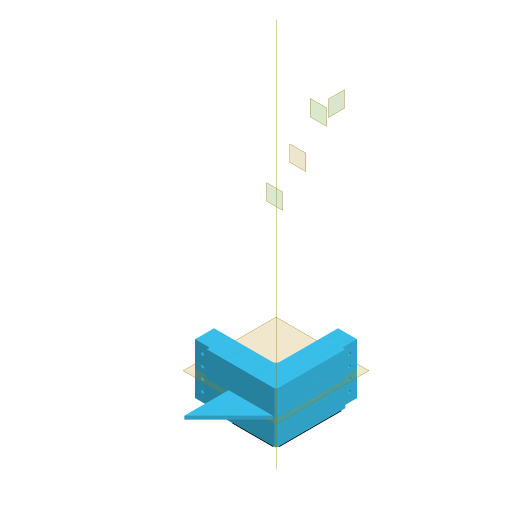
# Autodesk Inventor part: Столбик
Saved by Autodesk Inventor 2023.2 (Build 272271030, 271C)
## iProperties
Created: 2025-04-23
Part Number: Столбик
Material: Типовые
Document SubType Name: Modeling
Designer: Коноваленко
Density: 1 g/cm^3
Appearance: Бирюзовый
Author: Коноваленко
Autodesk Inventor part; units mm, degrees
ref_plane "YZ Plane" through (0, 0, 0) normal (1, 0, 0) x (0, 1, 0)
ref_plane "XY Plane" through (0, 0, 0) normal (0, 0, 1) x (1, 0, 0)
sketch "Эскиз1" plane through (0, 0, 0) normal (0, 1, 0) x (-1, 0, 0)
  line L0 (-30, -85) -> (-30, 30)
  line L1 (-30, 30) -> (85, 30)
  line L2 (85, 30) -> (85, 0)
  line L3 (85, 0) -> (0, 0)
  line L4 (0, 0) -> (0, -85)
  line L5 (0, -85) -> (-30, -85)
  circle A0 centre (-26, 26) radius 4
  line L6 (85, 26) -> (65, 26)
  line L7 (65, 26) -> (65, 30)
  circle A1 centre (5, -5) radius 5
  line L8 (-30, -85) -> (-26, -85)
  line L9 (-26, -85) -> (-26, -65)
  line L10 (-26, -65) -> (-30, -65)
  line L11 (-30, -65) -> (-30, -85)
  line L12 (0, -85) -> (-4, -85)
  line L13 (0, -65) -> (0, -85)
  line L14 (85, 0) -> (65, 0)
  line L15 (85, 4) -> (85, 0)
  point P0 (-26, 30)
  point P1 (-30, 26)
  point P2 (0, -5)
  point P3 (5, 0)
  dimension "d0" = 115
  dimension "d1" = 115
  dimension "d2" = 30
  dimension "d3" = 30
  dimension "d6" = 4
  dimension "d7" = 20
  dimension "d8" = 10
  dimension "d9" = 4
  dimension "d10" = 20
  dimension "d26" = 8
  constraints: 32 end point, 7 perpendicular, 4 horizontal, 4 point on line, 4 tangent, 2 centre point, 2 parallel, 1 vertical
  measures "d0" distance of L0.end L1.end
  measures "d1" distance of L0.start L0.end
  measures "d2" distance between parallel lines of L1 L3
  measures "d3" distance between parallel lines of L0 L4
  measures "d6" distance between parallel lines of L6 L1
  measures "d7" distance between parallel lines of L2 L7
  measures "d8" diameter of A1
  measures "d9" distance between parallel lines of L0 L9
  measures "d10" distance of L8.end L9.end
  measures "d26" diameter of A0
extrude "Выдавливание1" add sketch "Эскиз1" along normal blind 70 contours L0 A0 L1 L7 L6 L2 L3 L4 L5 L9 L10 | A0 | L4 L3 A1
sketch "Эскиз2" plane through (0, 0, 0) normal (0, -1, 0) x (1, 0, 0)
  line L0 (-5, 0) -> (-85, 0) projected
  line L1 (-30, 0) -> (-30, 30)
  line L2 (-30, 30) -> (26, 30)
  line L3 (30, 26) -> (30, -59)
  line L4 (0, -85) -> (0, -5) projected
  arc A0 (0, -5) -> (-5, 0) centre (-5, -5) ccw projected
  line L5 (0, -85) -> (0, -5) projected
  arc A1 (30, 26) -> (26, 30) centre (26, 26) ccw projected
  line L6 (30, -59) -> (0, -59)
  point P0 (0, 0)
  point P1 (-30, 15)
  point P2 (-65, 0)
  point P3 (0, -65)
  point P4 (0, -59)
  dimension "d134" = 60
  dimension "d135" = 30
  dimension "d136" = 30
  dimension "d137" = 85
  constraints: 8 end point, 4 perpendicular, 2 point on circle, 2 point on line, 1 midpoint
  measures "d134" distance between parallel lines of L3 L1
  measures "d135" distance between parallel lines of L0 L2
  measures "d136" distance between parallel lines of L4 L3
  measures "d137" distance of L3.start L3.end
sketch "Эскиз13" plane through (0, 70, 0) normal (0, 1, 0) x (1, 0, 0)
  line L0 (26, 65) -> (26, 85) projected
  line L1 (26, 85) -> (0, 85) projected
  line L2 (30, 65) -> (26, 65) projected
  line L3 (0, 30) -> (30, 30)
  line L4 (30, -26) -> (30, 65) projected
  line L5 (0, 85) -> (0, 5) projected
  point P0 (0, 0)
  point P1 (30, -30)
  dimension "d226" = 55
  constraints: 2 end point, 1 horizontal, 1 point on line
  measures "d226" distance between parallel lines of L1 L3
extrude "Выдавливание11" [suppressed]
ref_plane "РабПлоскость2" through (0, 300, -30) normal (0, 0, 1) x (1, 0, 0)
sketch "Эскиз16" plane through (0, 300, -30) normal (0, 0, 1) x (1, 0, 0)
  line L0 (7.5, 7) -> (22.5, 7)
  line L1 (22.5, 7) -> (20, 0)
  line L2 (7.5, 7) -> (10, 0)
  line L3 (30, -230) -> (30, 70) projected
  line L4 (10, 0) -> (20, 0)
  line L5 (30, -230) -> (30, 70) projected
  line L6 (0, 144) -> (0, -374) projected
  line L7 (30, -300) -> (30, -230) projected
  point P0 (96.6667, 0)
  dimension "d143" = 15
  dimension "d207" = 7
  dimension "d222" = 10
  dimension "d223" = 7.5
  dimension "d224" = 10
  constraints: 8 end point, 2 horizontal, 1 point on line
  measures "d143" distance of L0.start L0.end
  measures "d207" distance between parallel lines of L0 L4
  measures "d222" distance from line of L6 L2.end
  measures "d223" distance from line of L7 L0.end
  measures "d224" distance from line of L7 L1.end
extrude "Выдавливание13" [suppressed]
feature "Оболочка1" [suppressed]
fillet "Сопряжение6" [suppressed]
fillet "Сопряжение8" [suppressed]
sketch "Эскиз28" plane through (-80, 5, 0) normal (0, 1, 0) x (1, 0, 0)
  arc A0 (103, -25) -> (105, -23) centre (103, -23) ccw projected
  line L0 (105, -23) -> (105, 58) projected
  arc A1 (105, 58) -> (103, 60) centre (103, 58) ccw projected
  arc A2 (101, 62) -> (103, 60) centre (103, 62) ccw projected
  line L1 (101, 62) -> (101, 78) projected
  arc A3 (101, 78) -> (99, 80) centre (99, 78) ccw projected
  line L2 (99, 80) -> (80, 80) projected
  line L3 (80, 5) -> (80, 80) projected
  arc A4 (75, 0) -> (80, 5) centre (75, 5) ccw projected
  line L4 (0, 0) -> (75, 0) projected
  line L5 (0, 0) -> (0, -19) projected
  arc A5 (0, -19) -> (2, -21) centre (2, -19) ccw projected
  line L6 (2, -21) -> (18, -21) projected
  arc A6 (20, -23) -> (18, -21) centre (18, -23) ccw projected
  arc A7 (20, -23) -> (22, -25) centre (22, -23) ccw projected
  line L7 (22, -25) -> (103, -25) projected
  point P0 (80, 0)
extrude "Выдавливание19" [suppressed]
sketch "Эскиз27" plane through (-60, 10, 25) normal (0, 1, 0) x (1, 0, 0)
  circle A0 centre (75, 70) radius 3.1
  circle A1 centre (75, 40) radius 3.1
  circle A2 centre (75, 10) radius 3.1
  circle A3 centre (45, 10) radius 3.1
  circle A4 centre (15, 10) radius 3.1
  line L0 (83, 0) -> (2, 0) projected
  dimension "d231" = 17.945
  dimension "d234" = 10
  constraints: 5 centre point, 1 equal radius, 8 other
  measures "d234" distance from line of L0 A4.centre
ref_plane "РабПлоскость3" through (-80, 140, 0) normal (0, 1, 0) x (1, 0, 0)
sketch "Эскиз30" plane through (-80, 140, 0) normal (0, 1, 0) x (1, 0, 0)
  line L0 (103, -25) -> (22, -25) projected
  arc A0 (103, -25) -> (105, -23) centre (103, -23) ccw projected
  line L1 (105, 58) -> (105, -23) projected
  arc A1 (105, 58) -> (103, 60) centre (103, 58) ccw projected
  arc A2 (101, 62) -> (103, 60) centre (103, 62) ccw projected
  line L2 (101, 78) -> (101, 62) projected
  arc A3 (101, 78) -> (99, 80) centre (99, 78) ccw projected
  line L3 (80, 80) -> (99, 80) projected
  line L4 (80, 80) -> (80, 5) projected
  arc A4 (75, 0) -> (80, 5) centre (75, 5) ccw projected
  line L5 (75, 0) -> (0, 0) projected
  line L6 (0, -19) -> (0, 0) projected
  arc A5 (0, -19) -> (2, -21) centre (2, -19) ccw projected
  line L7 (18, -21) -> (2, -21) projected
  arc A6 (20, -23) -> (18, -21) centre (18, -23) ccw projected
  arc A7 (20, -23) -> (22, -25) centre (22, -23) ccw projected
  circle A8 centre (65, -15) radius 3.1 projected
  circle A9 centre (35, -15) radius 3.1 projected
  circle A10 centre (95, -15) radius 3.1 projected
  circle A11 centre (95, 15) radius 3.1 projected
  circle A12 centre (95, 45) radius 3.1 projected
  point P0 (80, 0)
extrude "Выдавливание20" [suppressed]
ref_plane "РабПлоскость4" through (-80, 150, 0) normal (0, -1, 0) x (1, 0, 0)
ref_plane "РабПлоскость5" through (-80, 100, 0) normal (0, 1, 0) x (1, 0, 0)
sketch "Эскиз31" plane through (-80, 100, 0) normal (0, 1, 0) x (1, 0, 0)
  arc A0 (103, 60) -> (101, 62) centre (103, 62) ccw projected
  arc A1 (105, 58) -> (103, 60) centre (103, 58) ccw projected
  line L0 (105, -23) -> (105, 58) projected
  arc A2 (103, -25) -> (105, -23) centre (103, -23) ccw projected
  line L1 (22, -25) -> (103, -25) projected
  arc A3 (20, -23) -> (22, -25) centre (22, -23) ccw projected
  arc A4 (18, -21) -> (20, -23) centre (18, -23) ccw projected
  line L2 (2, -21) -> (18, -21) projected
  arc A5 (0, -19) -> (2, -21) centre (2, -19) ccw projected
  line L3 (0, 0) -> (0, -19) projected
  line L4 (75, 0) -> (0, 0) projected
  line L5 (80, 80) -> (80, 5) projected
  line L6 (99, 80) -> (80, 80) projected
  arc A6 (101, 78) -> (99, 80) centre (99, 78) ccw projected
  line L7 (101, 62) -> (101, 78) projected
  arc A7 (75, 0) -> (80, 5) centre (75, 5) ccw projected
  point P0 (80, 0)
  constraints: 7 centre point
extrude "Выдавливание21" [suppressed]
pattern_linear "Прямоуг.массив1" [suppressed]
ref_plane "РабПлоскость8" through (-80, 200, 0) normal (0, 1, 0) x (1, 0, 0)
sketch "Эскиз33" plane through (-80, 200, 0) normal (0, 1, 0) x (1, 0, 0)
  arc A0 (101, 62) -> (103, 60) centre (103, 62) ccw projected
  line L0 (101, 78) -> (101, 62) projected
  line L1 (80, 80) -> (99, 80) projected
  line L2 (80, 80) -> (80, 5) projected
  line L3 (75, 0) -> (0, 0) projected
  line L4 (0, -19) -> (0, 0) projected
  line L5 (18, -21) -> (2, -21) projected
  arc A1 (20, -23) -> (18, -21) centre (18, -23) ccw projected
  line L6 (103, -25) -> (22, -25) projected
  line L7 (105, 58) -> (105, -23) projected
  arc A2 (20, -23) -> (22, -25) centre (22, -23) ccw projected
  arc A3 (20, -23) -> (22, -25) centre (22, -23) ccw projected
  arc A4 (0, -19) -> (2, -21) centre (2, -19) ccw projected
  arc A5 (0, -19) -> (2, -21) centre (2, -19) ccw projected
  arc A6 (103, -25) -> (105, -23) centre (103, -23) ccw projected
  arc A7 (103, -25) -> (105, -23) centre (103, -23) ccw projected
  arc A8 (75, 0) -> (80, 5) centre (75, 5) ccw projected
  arc A9 (101, 78) -> (99, 80) centre (99, 78) ccw projected
  arc A10 (105, 58) -> (103, 60) centre (103, 58) ccw projected
  arc A11 (105, 58) -> (103, 60) centre (103, 58) ccw projected
  arc A12 (20, -23) -> (22, -25) centre (22, -23) ccw projected
  arc A13 (20, -23) -> (22, -25) centre (22, -23) ccw projected
  arc A14 (20, -23) -> (22, -25) centre (22, -23) ccw projected
  arc A15 (20, -23) -> (22, -25) centre (22, -23) ccw projected
  arc A16 (20, -23) -> (22, -25) centre (22, -23) ccw projected
  arc A17 (20, -23) -> (22, -25) centre (22, -23) ccw projected
  arc A18 (0, -19) -> (2, -21) centre (2, -19) ccw projected
  arc A19 (0, -19) -> (2, -21) centre (2, -19) ccw projected
  arc A20 (0, -19) -> (2, -21) centre (2, -19) ccw projected
  arc A21 (0, -19) -> (2, -21) centre (2, -19) ccw projected
  arc A22 (0, -19) -> (2, -21) centre (2, -19) ccw projected
  arc A23 (0, -19) -> (2, -21) centre (2, -19) ccw projected
  arc A24 (103, -25) -> (105, -23) centre (103, -23) ccw projected
  arc A25 (103, -25) -> (105, -23) centre (103, -23) ccw projected
  arc A26 (103, -25) -> (105, -23) centre (103, -23) ccw projected
  arc A27 (103, -25) -> (105, -23) centre (103, -23) ccw projected
  arc A28 (103, -25) -> (105, -23) centre (103, -23) ccw projected
  arc A29 (103, -25) -> (105, -23) centre (103, -23) ccw projected
  arc A30 (101, 78) -> (99, 80) centre (99, 78) ccw projected
  arc A31 (101, 78) -> (99, 80) centre (99, 78) ccw projected
  arc A32 (101, 78) -> (99, 80) centre (99, 78) ccw projected
  arc A33 (101, 78) -> (99, 80) centre (99, 78) ccw projected
  arc A34 (101, 78) -> (99, 80) centre (99, 78) ccw projected
  arc A35 (101, 78) -> (99, 80) centre (99, 78) ccw projected
  arc A36 (101, 78) -> (99, 80) centre (99, 78) ccw projected
  arc A37 (105, 58) -> (103, 60) centre (103, 58) ccw projected
  arc A38 (105, 58) -> (103, 60) centre (103, 58) ccw projected
  arc A39 (105, 58) -> (103, 60) centre (103, 58) ccw projected
  arc A40 (105, 58) -> (103, 60) centre (103, 58) ccw projected
  arc A41 (105, 58) -> (103, 60) centre (103, 58) ccw projected
  arc A42 (105, 58) -> (103, 60) centre (103, 58) ccw projected
  point P0 (80, 0)
  point P1 (2, -21)
  point P2 (20, -23)
  point P3 (22, -25)
  constraints: 2 centre point
extrude "Выдавливание24" [suppressed]
pattern_linear "Прямоуг.массив2" [suppressed]
feature "Разделение3" [suppressed]
fillet "Сопряжение9" [suppressed]
fillet "Сопряжение10" [suppressed]
extrude "Выдавливание25" [suppressed]
ref_plane "РабПлоскость13" through (23, 363, -35) normal (0, 0, -1) x (-1, 0, 0)
sketch "Эскиз34" plane through (23, 363, -35) normal (0, 0, -1) x (-1, 0, 0)
  line L0 (7.595, -61) -> (8, -62.1339) projected
  line L1 (7.595, -61) -> (8, -62.1339) projected
  line L2 (8.405, -61) -> (7.595, -61) projected
  line L3 (8, -62.1339) -> (8.405, -61) projected
  point P0 (23, -363)
extrude "Выдавливание26" [suppressed]
sketch "Эскиз36" plane through (25, 57, 23) normal (-1, 0, 0) x (0, 0, 1)
  line L0 (-28, 38) -> (-101, 38) projected
  line L1 (-101, -2) -> (-28, -2) projected
  line L2 (-76, 38) -> (-71, 38)
  line L3 (-71, 38) -> (-71, -2)
  line L4 (-71, -2) -> (-76, -2)
  line L5 (-76, -2) -> (-76, 38)
  line L6 (-81, 0) -> (-81, 36) projected
  point P0 (-23, -57)
  point P1 (-76, -2)
  dimension "d264" = 14.559
  dimension "d270" = 5.467
  constraints: 8 end point, 2 parallel, 2 point on line, 1 horizontal, 1 perpendicular
extrude "Выдавливание27" [suppressed]
pattern_linear "Прямоуг.массив3" [suppressed]
ref_plane "РабПлоскость10" through (-85, 0, -85) normal (0.7071068, 0, -0.7071068) x (0, -1, 0)
mirror "Зеркальное отражение9" [suppressed]
ref_plane "РабПлоскость12" through (23, 293, 25) normal (0, 0, -1) x (-1, 0, 0)
sketch "Эскиз38" plane through (23, 293, 25) normal (0, 0, -1) x (-1, 0, 0)
  line L0 (64.282, 2) -> (76, 2)
  line L1 (76, 2) -> (76, -43)
  line L2 (76, -43) -> (64.282, -43)
  line L3 (64.282, -43) -> (64.282, 2)
  line L4 (83, 2) -> (85, 2) projected
  line L5 (81, 2) -> (81, -41) projected
  line L6 (28, -43) -> (101, -43) projected
  point P0 (23, -293)
  point P1 (84, 2)
  point P2 (70.141, -43)
  dimension "d279" = 11.718
  dimension "d301" = 5
  constraints: 8 end point, 2 midpoint, 2 parallel, 2 point on line, 1 horizontal, 1 perpendicular
  measures "d279" distance between parallel lines of L3 L1
  measures "d301" distance between parallel lines of L5 L1
extrude "Выдавливание29" [suppressed]
ref_plane "РабПлоскость11" through (25, 363, -58) normal (-1, 0, 0) x (0, 0, 1)
sketch "Эскиз40" plane through (25, 295, -35) normal (-1, 0, 0) x (0, 0, 1)
  line L0 (0, 0) -> (30, 0) projected
  line L1 (-23, -45) -> (58, -45) projected
  line L2 (-45, 70) -> (0, 70) projected
  line L3 (-18, 70) -> (-13, 70)
  line L4 (-13, -45) -> (-18, -45)
  line L5 (-45, 70) -> (-45, -43) projected
  line L6 (0, 0) -> (0, 70) projected
  line L7 (0, 40) -> (0, 35)
  line L8 (-45, 35) -> (-45, 40)
  line L9 (-45, 5) -> (-45, 0)
  line L10 (0, 0) -> (0, 5)
  line L11 (12, 0) -> (17, 0)
  line L12 (17, 0) -> (17, -45)
  line L13 (17, -45) -> (12, -45)
  line L14 (12, -45) -> (12, 0)
  line L15 (-43, -45) -> (30, -45) projected
  line L16 (-45, 40) -> (-18, 40)
  line L17 (-13, 40) -> (0, 40)
  line L18 (-18, 40) -> (-18, 70)
  line L19 (0, 35) -> (-13, 35)
  line L20 (-18, 35) -> (-45, 35)
  line L21 (-13, 70) -> (-13, 40)
  line L22 (0, 5) -> (-13, 5)
  line L23 (-18, 5) -> (-45, 5)
  line L24 (-18, -45) -> (-18, 0)
  line L25 (-18, 5) -> (-18, 35)
  line L26 (-45, 0) -> (-18, 0)
  line L27 (-13, 0) -> (0, 0)
  line L28 (-13, 35) -> (-13, 5)
  line L29 (-13, 0) -> (-13, -45)
  point P0 (35, -295)
  point P1 (15, 0)
  point P2 (14.5, -45)
  point P3 (12, 0)
  point P4 (17, 0)
  point P5 (-45, 5)
  point P6 (-45, 0)
  point P7 (-18, -45)
  point P8 (-13, -45)
  point P9 (0, 40)
  point P10 (-13, 70)
  point P11 (-45, 35)
  dimension "d312" = 7.296
  dimension "d313" = 53.553
  dimension "d314" = 30
  dimension "d315" = 13
  dimension "d316" = 5
  dimension "d317" = 5
  dimension "d318" = 5
  dimension "d319" = 5
  dimension "d320" = 5
  dimension "d321" = 5
  dimension "d322" = 5
  dimension "d323" = 45
  constraints: 48 end point, 22 parallel, 8 perpendicular, 6 horizontal, 6 point on line, 5 equal length, 3 midpoint
  measures "d314" distance of L3.end L17.start
  measures "d315" distance of L17.start L7.start
  measures "d316" distance between parallel lines of L21 L18
  measures "d317" distance between parallel lines of L28 L25
  measures "d318" distance between parallel lines of L29 L24
  measures "d319" distance between parallel lines of L22 L27
  measures "d320" distance between parallel lines of L17 L19
  measures "d321" distance between parallel lines of L20 L16
  measures "d322" distance between parallel lines of L26 L23
  measures "d323" distance of L27.start L4.start
pattern_linear "Прямоуг.массив6" [suppressed]
extrude "Выдавливание31" [suppressed]
fillet "Сопряжение12" [suppressed]
fillet "Сопряжение13" [suppressed]
fillet "Сопряжение14" [suppressed]
sketch "Эскиз41" plane through (25, 207, 23) normal (-1, 0, 0) x (0, 0, 1)
  line L0 (-101, 38) -> (-28, 38) projected
  line L1 (-81, -2) -> (0, -2) projected
  line L2 (-76, 38) -> (-71, 38)
  line L3 (-71, 38) -> (-71, -2)
  line L4 (-71, -2) -> (-76, -2)
  line L5 (-76, -2) -> (-76, 38)
  line L6 (-81, 0) -> (-81, 36) projected
  point P0 (-23, -207)
  point P1 (-76, -2)
  dimension "d329" = 9.532
  dimension "d330" = 2.688
  constraints: 8 end point, 2 parallel, 2 point on line, 1 horizontal, 1 perpendicular
extrude "Выдавливание32" [suppressed]
pattern_linear "Прямоуг.массив7" [suppressed]
mirror "Зеркальное отражение11" [suppressed]
fillet "Сопряжение15" [suppressed]
fillet "Сопряжение16" [suppressed]
fillet "Сопряжение17" [suppressed]
sketch "Эскиз42" plane through (25, 160, -58) normal (-1, 0, 0) x (0, 0, 1)
  line L0 (-22, 0) -> (53, 0) projected
  line L1 (-20, 40) -> (53, 40) projected
  line L2 (29.5, 0) -> (26.5, 0)
  line L3 (26.5, 0) -> (26.5, 40)
  line L4 (26.5, 40) -> (29.5, 40)
  line L5 (29.5, 40) -> (29.5, 0)
  line L6 (-22, 0) -> (-22, 38) projected
  point P0 (58, -160)
  point P1 (26.5, 0)
  dimension "d339" = 9.768
  dimension "d340" = 45.54
  constraints: 8 end point, 2 parallel, 2 point on line, 1 horizontal, 1 perpendicular
extrude "Выдавливание33" [suppressed]
pattern_linear "Прямоуг.массив8" [suppressed]
mirror "Зеркальное отражение12" [suppressed]
fillet "Сопряжение18" [suppressed]
fillet "Сопряжение19" [suppressed]
fillet "Сопряжение20" [suppressed]
sketch "Эскиз43" plane through (25, 140, -58) normal (-1, 0, 0) x (0, 0, 1)
  line L0 (-22, 0) -> (53, 0) projected
  line L1 (-20, -40) -> (53, -40) projected
  line L2 (26.5, 0) -> (29.5, 0)
  line L3 (29.5, 0) -> (29.5, -40)
  line L4 (29.5, -40) -> (26.5, -40)
  line L5 (26.5, -40) -> (26.5, 0)
  line L6 (-22, -38) -> (-22, 0) projected
  point P0 (58, -140)
  dimension "d349" = 4.923
  dimension "d350" = 48.122
  constraints: 8 end point, 2 parallel, 2 point on line, 1 horizontal, 1 perpendicular
extrude "Выдавливание34" [suppressed]
fillet "Сопряжение21" [suppressed]
pattern_linear "Прямоуг.массив9" [suppressed]
mirror "Зеркальное отражение13" [suppressed]
fillet "Сопряжение22" [suppressed]
fillet "Сопряжение23" [suppressed]
fillet "Сопряжение24" [suppressed]
ref_plane "РабПлоскость14" through (-80, 75, 0) normal (0, -1, 0) x (1, 0, 0)
mirror "Зеркальное отражение14" [suppressed]
fillet "Сопряжение25" [suppressed]
fillet "Сопряжение26" [suppressed]
fillet "Сопряжение27" [suppressed]
sketch "Эскиз44" plane through (-80, 75, 0) normal (0, -1, 0) x (1, 0, 0)
  line L0 (42.8482, 31) -> (106.6, 31)
  line L1 (106.6, 31) -> (46, 91.6)
  line L2 (46, 91.6) -> (46, 31)
  line L3 (46, 31) -> (42.8482, 31)
  line L4 (15, 30) -> (106, 30) projected
  line L5 (110, 26) -> (110, -65) projected
  line L6 (15, 30) -> (106, 30) projected
  line L7 (106, 30) -> (105, 31)
  line L8 (103.5858, 31) -> (104.5858, 30)
  point P0 (80, 0)
  point P1 (105.5, 30.5)
  point P2 (105, 30)
  dimension "d363" = 31.67
  dimension "d364" = 12.403
  dimension "d367" = 0.745
  dimension "d368" = 77.702
  constraints: 13 end point, 6 point on line, 2 parallel, 1 collinear, 1 horizontal, 1 midpoint, 1 perpendicular
extrude "Выдавливание35" [suppressed]
extrude "Выдавливание36" [suppressed]
pattern_linear "Прямоуг.массив10" [suppressed]
sketch "Эскиз46" plane through (-80, 10, 0) normal (0, 1, 0) x (1, 0, 0)
  line L0 (18, -21) -> (2, -21) projected
  line L1 (18, -21) -> (18, 0)
  line L2 (75, 0) -> (0, 0) projected
  arc A0 (0, -19) -> (2, -21) centre (2, -19) ccw projected
  line L3 (0, -19) -> (0, 0) projected
  point P0 (80, 0)
  constraints: 2 end point, 1 point on line, 1 vertical
extrude "Выдавливание38" [suppressed]
sketch "Эскиз45" plane through (-85, 0, 26) normal (0, 0, 1) x (1, 0, 0)
  circle A0 centre (10, 133.884) radius 6.3785
  line L0 (0, 150) -> (20, 150) projected
  line L1 (10, 150) -> (10, 100.3014) construction
  circle A1 centre (10, 93.884) radius 6.3785
  circle A2 centre (10, 53.884) radius 6.3785
  circle A3 centre (10, 13.884) radius 6.3785
  point P0 (85, 0)
  dimension "d377" = 12.757
  dimension "d378" = 16.116
  dimension "d381" = 40
  constraints: 4 centre point, 2 end point, 2 vertical, 1 midpoint, 1 point on line, 6 other
  measures "d377" diameter of A0
  measures "d378" distance from line of A0.centre L0
  measures "d381" distance of A0.centre A1.centre
extrude "Выдавливание37" [suppressed]
mirror "Зеркальное отражение16" [suppressed]
mirror "Зеркальное отражение15" [suppressed]
sketch "Эскиз48" plane through (0, 0, 0) normal (0, -1, 0) x (1, 0, 0)
  line L0 (26, -65) -> (26, -85) projected
  line L1 (26, -85) -> (0, -85) projected
  line L2 (30, 26) -> (30, -65) projected
  line L3 (30, -65) -> (26, -65) projected
  line L4 (0, -62) -> (0, -55) projected
  line L5 (0, -85) -> (0, -5) projected
  line L6 (30, -58.5) -> (0, -58.5)
  line L7 (-46, 0) -> (-25, 0) projected
  line L8 (-65, 30) -> (26, 30) projected
  line L9 (-41.455, 30) -> (-41.455, 0)
  line L10 (-85, 0) -> (-85, 26) projected
  line L11 (-65, 26) -> (-65, 30) projected
  line L12 (-85, 26) -> (-65, 26) projected
  line L13 (-5, 0) -> (-85, 0) projected
  point P0 (0, 0)
  point P1 (13, -85)
  point P2 (0, -58.5)
  dimension "d393" = 26.5
  dimension "d396" = 43.545
  constraints: 4 end point, 4 point on line, 1 midpoint, 1 perpendicular, 1 vertical
  measures "d393" distance from line of point (13, -85) L6
  measures "d396" distance between parallel lines of L10 L9
extrude "Выдавливание40" [suppressed]
ref_plane "РабПлоскость15" through (-65, 225, 30) normal (0, -1, 0) x (1, 0, 0)
sketch "Эскиз50" plane through (-65, 225, 30) normal (0, -1, 0) x (1, 0, 0)
  line L0 (31, 61.6) -> (31, 1)
  line L1 (91.6, 1) -> (31, 61.6)
  line L2 (31, 1) -> (91.6, 1)
  line L3 (91, 0) -> (90, 1)
  line L4 (88.5858, 1) -> (89.5858, 0)
  line L5 (0, 0) -> (91, 0) projected
  point P0 (65, -30)
  dimension "d399" = 60.6
  dimension "d400" = 1
  dimension "d401" = 45
  dimension "d402" = 1
  constraints: 10 end point
  measures "d399" distance of L0.start L0.end
  measures "d400" distance between parallel lines of L5 L2
  measures "d401" angle of L1 L2
  measures "d402" distance between parallel lines of L3 L4
extrude "Выдавливание41" [suppressed]
extrude "Выдавливание42" [suppressed]
pattern_linear "Прямоуг.массив11" [suppressed]
sketch "Эскиз51" plane through (-85, 70, 26) normal (0, 0, 1) x (1, 0, 0)
  line L0 (0, 0) -> (20, 0) projected
  line L1 (10, 0) -> (10, -150) construction
  line L2 (80, -150) -> (0, -150) projected
  circle A0 centre (10, -6.368) radius 4.958
  circle A1 centre (10, -46.368) radius 4.958
  circle A2 centre (10, -86.368) radius 4.958
  circle A3 centre (10, -126.368) radius 4.958
  point P0 (85, -70)
  dimension "d408" = 9.916
  dimension "d409" = 6.368
  dimension "d412" = 40
  constraints: 4 centre point, 2 end point, 2 point on line, 2 vertical, 1 midpoint, 6 other
  measures "d408" diameter of A0
  measures "d409" distance from line of L0 A0.centre
  measures "d412" distance of A0.centre A1.centre
sketch "Эскиз52" plane through (-80, 160, 0) normal (0, 1, 0) x (1, 0, 0)
  line L0 (18, -21) -> (2, -21) projected
  line L1 (18, -21) -> (18, 0)
  line L2 (75, 0) -> (0, 0) projected
  arc A0 (0, -19) -> (2, -21) centre (2, -19) ccw projected
  line L3 (0, -19) -> (0, 0) projected
  point P0 (80, 0)
  constraints: 2 end point, 1 point on line, 1 vertical
extrude "Выдавливание43" [suppressed]
extrude "Выдавливание44" [suppressed]
mirror "Зеркальное отражение17" [suppressed]
sketch "Эскиз54" plane through (0, 300, -55) normal (0, 1, 0) x (1, 0, 0)
  line L0 (19, 7) -> (0, 7)
  line L1 (0, 23) -> (0, 0) projected
  line L2 (0, 25) -> (0, 23) projected
  line L3 (19, 25) -> (0, 25) projected
  arc A0 (21, 23) -> (19, 25) centre (19, 23) ccw projected
  line L4 (21, 7) -> (21, 23) projected
  line L5 (19, 7) -> (21, 7) projected
  point P0 (0, -55)
  constraints: 2 end point, 1 horizontal, 1 point on line
extrude "Выдавливание46" [suppressed]
sketch "Эскиз55" plane through (26, 370, -65) normal (1, 0, 0) x (0, 0, -1)
  circle A0 centre (10, -45) radius 2
  circle A1 centre (10, -85) radius 2 projected
  line L0 (20, -220) -> (20, 0) projected
  point P0 (-65, -370)
  dimension "d427" = 5.972
  dimension "d428" = 22.239
  dimension "d429" = 12.1
  constraints: 1 centre point
extrude "Выдавливание47" [suppressed]
ref_plane "РабПлоскость16" through (0, 335, -46) normal (0, 1, 0) x (1, 0, 0)
sketch "Эскиз56" plane through (0, 335, -46) normal (0, 1, 0) x (1, 0, 0)
  line L0 (0, -17) -> (86.6, -17)
  line L1 (86.6, -17) -> (0, -103.6)
  line L2 (0, -103.6) -> (0, -17)
  line L3 (0, -16) -> (30, -16) projected
  line L4 (0, -16) -> (0, -41) projected
  line L5 (0, -17) -> (1.3333, -16)
  line L6 (10, -16) -> (0, -16) projected
  line L7 (3, -16) -> (1.6667, -17)
  line L8 (31, -17) -> (41, -17)
  line L9 (41, -17) -> (41, 42.6177)
  line L10 (41, 42.6177) -> (31, 42.6177)
  line L11 (31, 42.6177) -> (31, -17)
  line L12 (30, -16) -> (30, 19) projected
  line L13 (30, -16) -> (31, -17)
  line L14 (30, -72) -> (30, 19) projected
  line L15 (30, -15.2023) -> (31, -16.168)
  point P0 (0, -46)
  point P1 (26.6, -77)
  dimension "d432" = 42.29
  dimension "d433" = 4.799
  dimension "d434" = 0.546
  dimension "d436" = 4.757
  dimension "d444" = 3.802
  dimension "d445" = 6.685
  dimension "d446" = 6.42
  constraints: 22 end point, 11 point on line, 3 parallel, 2 horizontal, 2 perpendicular
extrude "Выдавливание48" [suppressed]
extrude "Выдавливание49" [suppressed]
pattern_linear "Прямоуг.массив12" [suppressed]
extrude "Выдавливание50" [suppressed]
fillet "Сопряжение28" [suppressed]
extrude "Выдавливание51" [suppressed]
pattern_linear "Прямоуг.массив13" [suppressed]
pattern_linear "Прямоуг.массив14" [suppressed]
shell "Оболочка2" thickness 5 removed faces 3 at (-0.8688, 46.6667, -2.1834) at (0, 23.3333, -58.3333) at (-31.6667, 23.3333, 0)
sketch "Эскиз57" plane through (-60, 5, 25) normal (0, 1, 0) x (1, 0, 0)
  line L0 (85, 85) -> (81, 85) projected
  line L1 (60, 30) -> (60, 105) projected
  line L2 (-20, 4) -> (0, 4) projected
  line L3 (-20, 25) -> (55, 25) projected
  line L4 (-20, 25) -> (-20, 4) projected
  line L5 (81, 105) -> (60, 105) projected
  line L6 (81, 85) -> (81, 105) projected
  line L7 (-2, 4) -> (-2, 25)
  line L8 (81, 87) -> (60, 87)
  point P0 (60, 25)
  dimension "d469" = 18
  dimension "d471" = 18
  constraints: 4 end point, 4 point on line, 2 perpendicular
  measures "d469" distance between parallel lines of L4 L7
  measures "d471" distance between parallel lines of L8 L5
extrude "Выдавливание52" add sketch "Эскиз57" along normal up to surface (60 mm away)
ref_plane "РабПлоскость17" through (-60, 35, 25) normal (0, 1, 0) x (1, 0, 0)
sketch "Эскиз60" plane through (-60, 35, 25) normal (0, 1, 0) x (1, 0, 0)
  line L0 (-2, 25) -> (-2, 4) projected
  line L1 (-2, 4) -> (0, 4) projected
  line L2 (0, 4) -> (0, 0) projected
  line L3 (0, 0) -> (85, 0) projected
  line L4 (85, 0) -> (85, 85) projected
  line L5 (85, 85) -> (81, 85) projected
  line L6 (81, 85) -> (81, 87) projected
  line L7 (81, 87) -> (60, 87) projected
  line L8 (60, 30) -> (60, 87) projected
  arc A0 (55, 25) -> (60, 30) centre (55, 30) ccw projected
  line L9 (-2, 25) -> (55, 25) projected
  point P0 (60, 25)
extrude "Выдавливание53" add sketch "Эскиз60" along normal mid plane 5
sketch "Эскиз61" plane through (25, 5, -60) normal (-1, 0, 0) x (0, 0, 1)
  line L0 (85, 27.5) -> (0, 27.5) projected
  line L1 (55, 0) -> (-2, 0) projected
  line L2 (28.5, 27.5) -> (31.5, 27.5)
  line L3 (31.5, 27.5) -> (31.5, 0)
  line L4 (31.5, 0) -> (28.5, 0)
  line L5 (28.5, 0) -> (28.5, 27.5)
  line L6 (-2, 0) -> (-2, 27.5) projected
  point P0 (60, -5)
  point P1 (28.5, 0)
  dimension "d474" = 3
  dimension "d475" = 30.5
  constraints: 8 end point, 2 parallel, 2 point on line, 1 horizontal, 1 perpendicular
  measures "d474" distance between parallel lines of L3 L5
  measures "d475" distance between parallel lines of L6 L5
extrude "Выдавливание54" add sketch "Эскиз61" along normal blind 10
pattern_linear "Прямоуг.массив15" count 2 spacing 30 along (0, 0, 1) of "Выдавливание54"
mirror "Зеркальное отражение18" about plane through (-85, 0, -85) normal (0.7071068, 0, -0.7071068) of "Выдавливание54", "Прямоуг.массив15"
mirror "Зеркальное отражение19" about plane through (-60, 35, 25) normal (0, 1, 0) of "Выдавливание54", "Прямоуг.массив15", "Зеркальное отражение18"
fillet "Сопряжение29" radius 2 50 edges at (25, 37.5, -45.75) (25, 65, -45.75) (25, 65, -15) (25, 37.5, -15) (25, 37.5, 13.25) (25, 65, 13.25) (13.25, 37.5, 25) (25, 51.25, 25) (13.25, 65, 25) (-15, 65, 25) (-15, 37.5, 25) (-45.75, 37.5, 25) (-45.75, 65, 25) (-62, 37.5, 10.5) (-62, 65, 10.5) (10.5, 37.5, -62) (10.5, 65, -62) (21, 51.25, -60) (25, 51.25, -60) (-60, 51.25, 21) (-60, 51.25, 25) (25, 51.25, -31.5) (20, 37.5, -31.5) (15, 37.5, -30) (20, 65, -31.5) (15, 65, -30) (15, 65, 0) (20, 65, -1.5) (25, 51.25, -1.5) (20, 37.5, -1.5) (15, 37.5, 0) (0, 37.5, 15) (-1.5, 37.5, 20) (-1.5, 51.25, 25) (-1.5, 65, 20) (0, 65, 15) (-30, 65, 15) (-31.5, 65, 20) (-31.5, 51.25, 25) (-31.5, 37.5, 20) (-30, 37.5, 15) (-28.5, 37.5, 20) (-28.5, 51.25, 25) (-28.5, 65, 20) (20, 37.5, -28.5) (25, 51.25, -28.5) (20, 65, -28.5) (25, 32.5, -45.75) (20, 32.5, -31.5) (15, 32.5, -30)
fillet "Сопряжение30" radius 2 32 edges at (24.4142, 31.9142, -32.0858) (25, 17.75, -31.5) (20, 5, -31.5) (15, 5, -30) (20, 5, -28.5) (25, 17.75, -28.5) (18, 32.5, -28.5) (10.5, 32.5, -62) (-62, 32.5, 10.5) (-45.75, 32.5, 25) (-31.5, 5, 20) (-31.5, 18.75, 25) (-31.5, 32.5, 20) (-28.5, 5, 20) (-28.5, 18.75, 25) (-28.5, 32.5, 20) (-30, 32.5, 15) (-15, 32.5, 25) (13.25, 32.5, 25) (0, 32.5, 15) (-1.5, 32.5, 20) (-1.5, 18.75, 25) (-1.5, 5, 20) (0, 5, 15) (20, 5, -1.5) (15, 5, 0) (25, 18.75, 25) (25, 32.5, 13.25) (25, 32.5, -14) (25, 18.75, -1.5) (20, 32.5, -1.5) (15, 32.5, 0)
fillet "Сопряжение31" radius 2 9 edges at (1.5, 64.4142, 24.4142) (1.5, 65, 18) (1.5, 38.0858, 24.4142) (1.5, 37.5, 18) (1.5, 51.25, 25) (1.5, 31.9142, 24.4142) (1.5, 32.5, 18) (1.5, 17.75, 25) (1.5, 5, 19)
fillet "Сопряжение32" radius 2 9 edges at (24.4142, 38.0858, 1.5) (25, 51.25, 1.5) (24.4142, 64.4142, 1.5) (18, 65, 1.5) (18, 37.5, 1.5) (18, 32.5, 1.5) (25, 17.75, 1.5) (24.4142, 31.9142, 1.5) (19, 5, 1.5)
sketch "Эскиз62" plane through (-85, 0, 26) normal (0, 0, 1) x (1, 0, 0)
  line L0 (80, 70) -> (0, 70) projected
  line L1 (10, 70) -> (10, 0) construction
  line L2 (80, 0) -> (0, 0) projected
  line L3 (0, 0) -> (0, 70) projected
  circle A0 centre (10, 57.5) radius 2
  circle A1 centre (10, 42.5) radius 2
  circle A2 centre (10, 27.5) radius 2
  circle A3 centre (10, 12.5) radius 2
  point P0 (85, 0)
  dimension "d485" = 10
  dimension "d486" = 4
  dimension "d487" = 12.5
  dimension "d488" = 15
  dimension "d489" = 15
  dimension "d490" = 15
  constraints: 6 point on line, 4 centre point, 3 equal radius, 2 end point, 1 vertical
  measures "d485" distance between parallel lines of L3 L1
  measures "d486" diameter of A0
  measures "d487" distance from line of L0 A0.centre
  measures "d488" distance of A1.centre A0.centre
  measures "d489" distance of A1.centre A2.centre
  measures "d490" distance of A3.centre A2.centre
extrude "Выдавливание55" cut sketch "Эскиз62" against normal up to surface (26 mm away)
mirror "Зеркальное отражение20" about plane through (-85, 0, -85) normal (0.7071068, 0, -0.7071068) of "Выдавливание55"
sketch "Эскиз63" plane through (-62, 5, 0) normal (0, 1, 0) x (1, 0, 0)
  circle A0 centre (77, 45) radius 3.1
  circle A1 centre (77, 15) radius 3.1
  circle A2 centre (77, -15) radius 3.1
  circle A3 centre (47, -15) radius 3.1
  circle A4 centre (17, -15) radius 3.1
  point P0 (62, 0)
  constraints: 5 centre point, 10 other
extrude "Выдавливание56" cut sketch "Эскиз63" against normal up to surface (5 mm away)
sketch "Эскиз64" plane through (-60, 35, 25) normal (0, 1, 0) x (1, 0, 0)
  line L0 (26, -6) -> (86.6, -6)
  line L1 (86.6, -6) -> (26, -66.6)
  line L2 (26, -66.6) -> (26, -6)
  line L3 (-5, -5) -> (86, -5) projected
  line L4 (-5, -5) -> (86, -5) projected
  arc A0 (86, -5) -> (90, -1) centre (86, -1) ccw projected
  line L5 (86, -5) -> (85.5833, -6)
  line L6 (84.9167, -5) -> (84.5, -6)
  point P0 (60, 25)
  dimension "d495" = 45
  dimension "d496" = 60.6
  dimension "d497" = 1
  dimension "d498" = 0.6
  dimension "d499" = 1
  constraints: 10 end point, 3 point on line, 1 coincident, 1 horizontal, 1 parallel, 1 perpendicular
  measures "d495" angle of L1 L0
  measures "d496" distance of L1.end L0.start
  measures "d497" distance between parallel lines of L3 L0
  measures "d498" horizontal distance of L0.end point (86, -5)
  measures "d499" distance between parallel lines of L5 L6
extrude "Выдавливание57" add sketch "Эскиз64" along normal mid plane 5 contours L0 L1 L2
extrude "Выдавливание58" add sketch "Эскиз64" along normal mid plane 2 contours L6 L3 L5 L0
pattern_linear "Прямоуг.массив16" count 6 spacing 10 along (-1, 0, 0) of "Выдавливание58"
